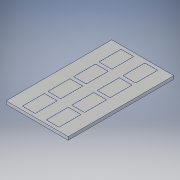
# Autodesk Inventor part: Assembly Plate
Saved by Autodesk Inventor 2019.4 (Build 234330000, 330)
## iProperties
Created: 2021-01-11
Part Number: Assembly Plate
Material: Aluminum 6061
Document SubType Name: Modeling
Designer: caleb
Density: 2.7 g/cm^3
Appearance: Aluminum - Flat
Author: caleb
Autodesk Inventor part; units mm, degrees
ref_plane "YZ Plane" through (0, 0, 0) normal (1, 0, 0) x (0, 1, 0)
ref_plane "XZ Plane" through (0, 0, 0) normal (0, 1, 0) x (-1, 0, 0)
ref_plane "XY Plane" through (0, 0, 0) normal (0, 0, 1) x (1, 0, 0)
sketch "Sketch1" plane through (0, 0, 0) normal (0, 1, 0) x (-1, 0, 0)
  line L0 (-63.5, 107.95) -> (63.5, 107.95)
  line L1 (63.5, 107.95) -> (63.5, -107.95)
  line L2 (63.5, -107.95) -> (-63.5, -107.95)
  line L3 (-63.5, -107.95) -> (-63.5, 107.95)
  line L4 (-63.5, 107.95) -> (63.5, -107.95) construction
  line L5 (63.5, 107.95) -> (-63.5, -107.95) construction
  point P0 (0, 0)
  dimension "d0" = 127
  dimension "d1" = 215.9
  constraints: 12 end point, 2 midpoint, 2 parallel, 1 horizontal, 1 perpendicular
  measures "d0" distance of L1.end L2.end
  measures "d1" distance of L0.end L1.end
extrude "Extrusion1" add sketch "Sketch1" along normal blind 6.35
sketch "Sketch7" plane through (0, 6.35, 0) normal (0, 1, 0) x (1, 0, 0)
  line L0 (-36.838, -100.75) -> (-11.838, -100.75)
  line L1 (-11.338, -100.25) -> (-11.338, -56.25)
  line L2 (-11.838, -55.75) -> (-36.838, -55.75)
  line L3 (-37.338, -56.25) -> (-37.338, -100.25)
  line L4 (-63.5, -107.95) -> (63.5, -107.95) projected
  line L5 (-63.5, 107.95) -> (-63.5, -107.95) projected
  arc A0 (-36.838, -55.75) -> (-37.338, -56.25) centre (-36.838, -56.25) ccw
  arc A1 (-11.338, -56.25) -> (-11.838, -55.75) centre (-11.838, -56.25) ccw
  arc A2 (-11.838, -100.75) -> (-11.338, -100.25) centre (-11.838, -100.25) ccw
  arc A3 (-37.338, -100.25) -> (-36.838, -100.75) centre (-36.838, -100.25) ccw
  arc A4 (-11.838, -48.55) -> (-11.338, -48.05) centre (-11.838, -48.05) ccw
  arc A5 (-37.338, -48.05) -> (-36.838, -48.55) centre (-36.838, -48.05) ccw
  line L6 (-11.338, -48.05) -> (-11.338, -4.05)
  line L7 (-37.338, -4.05) -> (-37.338, -48.05)
  line L8 (-11.838, -3.55) -> (-36.838, -3.55)
  arc A6 (-36.838, -3.55) -> (-37.338, -4.05) centre (-36.838, -4.05) ccw
  arc A7 (-11.338, -4.05) -> (-11.838, -3.55) centre (-11.838, -4.05) ccw
  line L9 (-36.838, -48.55) -> (-11.838, -48.55)
  arc A8 (-11.838, 3.65) -> (-11.338, 4.15) centre (-11.838, 4.15) ccw
  arc A9 (-37.338, 4.15) -> (-36.838, 3.65) centre (-36.838, 4.15) ccw
  line L10 (-11.338, 4.15) -> (-11.338, 48.15)
  line L11 (-37.338, 48.15) -> (-37.338, 4.15)
  line L12 (-11.838, 48.65) -> (-36.838, 48.65)
  arc A10 (-36.838, 48.65) -> (-37.338, 48.15) centre (-36.838, 48.15) ccw
  arc A11 (-11.338, 48.15) -> (-11.838, 48.65) centre (-11.838, 48.15) ccw
  line L13 (-36.838, 3.65) -> (-11.838, 3.65)
  arc A12 (-11.838, 55.85) -> (-11.338, 56.35) centre (-11.838, 56.35) ccw
  arc A13 (-37.338, 56.35) -> (-36.838, 55.85) centre (-36.838, 56.35) ccw
  line L14 (-11.338, 56.35) -> (-11.338, 100.35)
  line L15 (-37.338, 100.35) -> (-37.338, 56.35)
  line L16 (-11.838, 100.85) -> (-36.838, 100.85)
  arc A14 (-36.838, 100.85) -> (-37.338, 100.35) centre (-36.838, 100.35) ccw
  arc A15 (-11.338, 100.35) -> (-11.838, 100.85) centre (-11.838, 100.35) ccw
  line L17 (-36.838, 55.85) -> (-11.838, 55.85)
  arc A16 (36.822, -100.75) -> (37.322, -100.25) centre (36.822, -100.25) ccw
  arc A17 (11.322, -100.25) -> (11.822, -100.75) centre (11.822, -100.25) ccw
  line L18 (37.322, -100.25) -> (37.322, -56.25)
  line L19 (11.322, -56.25) -> (11.322, -100.25)
  line L20 (36.822, -55.75) -> (11.822, -55.75)
  arc A18 (11.822, -55.75) -> (11.322, -56.25) centre (11.822, -56.25) ccw
  arc A19 (37.322, -56.25) -> (36.822, -55.75) centre (36.822, -56.25) ccw
  line L21 (11.822, -100.75) -> (36.822, -100.75)
  arc A20 (36.822, -48.55) -> (37.322, -48.05) centre (36.822, -48.05) ccw
  arc A21 (11.322, -48.05) -> (11.822, -48.55) centre (11.822, -48.05) ccw
  line L22 (37.322, -48.05) -> (37.322, -4.05)
  line L23 (11.322, -4.05) -> (11.322, -48.05)
  line L24 (36.822, -3.55) -> (11.822, -3.55)
  arc A22 (11.822, -3.55) -> (11.322, -4.05) centre (11.822, -4.05) ccw
  arc A23 (37.322, -4.05) -> (36.822, -3.55) centre (36.822, -4.05) ccw
  line L25 (11.822, -48.55) -> (36.822, -48.55)
  arc A24 (36.822, 3.65) -> (37.322, 4.15) centre (36.822, 4.15) ccw
  arc A25 (11.322, 4.15) -> (11.822, 3.65) centre (11.822, 4.15) ccw
  line L26 (37.322, 4.15) -> (37.322, 48.15)
  line L27 (11.322, 48.15) -> (11.322, 4.15)
  line L28 (36.822, 48.65) -> (11.822, 48.65)
  arc A26 (11.822, 48.65) -> (11.322, 48.15) centre (11.822, 48.15) ccw
  arc A27 (37.322, 48.15) -> (36.822, 48.65) centre (36.822, 48.15) ccw
  line L29 (11.822, 3.65) -> (36.822, 3.65)
  arc A28 (36.822, 55.85) -> (37.322, 56.35) centre (36.822, 56.35) ccw
  arc A29 (11.322, 56.35) -> (11.822, 55.85) centre (11.822, 56.35) ccw
  line L30 (37.322, 56.35) -> (37.322, 100.35)
  line L31 (11.322, 100.35) -> (11.322, 56.35)
  line L32 (36.822, 100.85) -> (11.822, 100.85)
  arc A30 (11.822, 100.85) -> (11.322, 100.35) centre (11.822, 100.35) ccw
  arc A31 (37.322, 100.35) -> (36.822, 100.85) centre (36.822, 100.35) ccw
  line L33 (11.822, 55.85) -> (36.822, 55.85)
  line L34 (63.5, -107.95) -> (63.5, 107.95) projected
  point P0 (0, 0)
  point P1 (-37.338, -100.75)
  point P2 (-11.338, -100.75)
  point P3 (-37.338, -55.75)
  point P4 (-37.338, -48.55)
  point P5 (-11.338, -48.55)
  point P6 (-37.338, -3.55)
  point P7 (-37.338, 3.65)
  point P8 (-11.338, 3.65)
  point P9 (-37.338, 48.65)
  point P10 (-37.338, 55.85)
  point P11 (-11.338, 55.85)
  point P12 (-37.338, 100.85)
  point P13 (11.322, -100.75)
  point P14 (37.322, -100.75)
  point P15 (11.322, -55.75)
  point P16 (11.322, -48.55)
  point P17 (37.322, -48.55)
  point P18 (11.322, -3.55)
  point P19 (11.322, 3.65)
  point P20 (37.322, 3.65)
  point P21 (11.322, 48.65)
  point P22 (11.322, 55.85)
  point P23 (37.322, 55.85)
  point P24 (11.322, 100.85)
  dimension "d76" = 45
  dimension "d77" = 26
  dimension "d78" = 7.2
  dimension "d79" = 26.162
  dimension "d80" = 0.5
  dimension "d83" = 52.2
  dimension "d86" = 48.66
  dimension "d91" = 26.178
  constraints: 64 end point, 64 point on circle, 48 point on line, 32 centre point, 8 tangent, 3 equal radius, 2 horizontal, 2 parallel, 1 perpendicular, 1 vertical, 161 other
  measures "d76" distance of point (-37.338, -55.75) point (-37.338, -100.75)
  measures "d77" distance of point (-37.338, -100.75) point (-11.338, -100.75)
  measures "d78" distance between parallel lines of L4 L0
  measures "d79" distance between parallel lines of L5 L3
  measures "d80" radius of A0
  measures "d83" distance of A2.centre A4.centre
  measures "d86" distance of A2.centre A16.centre
  measures "d91" distance between parallel lines of L34 L18
extrude "Extrusion6" cut sketch "Sketch7" against normal blind 0.1
body "Solid1"
